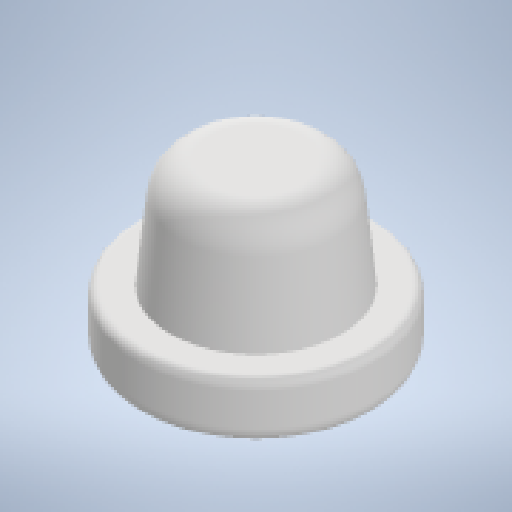
# Autodesk Inventor part: Part5
Saved by Autodesk Inventor 2025.1 (Build 291241000, 241)
## iProperties
Created: 2025-02-27
Part Number: Part5
Material: Generic
Document SubType Name: Modeling
Designer: santiago
Density: 1 g/cm^3
Appearance: Default
Author: santiago
Autodesk Inventor part; units mm, degrees
ref_plane "YZ Plane" through (0, 0, 0) normal (1, 0, 0) x (0, 1, 0)
ref_plane "XZ Plane" through (0, 0, 0) normal (0, 1, 0) x (-1, 0, 0)
ref_plane "XY Plane" through (0, 0, 0) normal (0, 0, 1) x (1, 0, 0)
sketch "Sketch1" plane through (0, 0, 0) normal (1, 0, 0) x (0, 1, 0)
  line L0 (10, 0) -> (10, 4.5)
  line L1 (10, 4.5) -> (2.5, 5.2)
  line L2 (2.5, 5.2) -> (2.5, 7.2)
  line L3 (2.5, 7.2) -> (0, 7.2)
  line L4 (0, 7.2) -> (0, 0)
  line L5 (10, 0) -> (0, 0)
  dimension "d0" = 4.5
  dimension "d1" = 10
  dimension "d2" = 2.5
  dimension "d3" = 2
  dimension "d5" = 7.2
  dimension "d6" = 5.2
  constraints: 12 end point, 2 perpendicular, 1 horizontal, 1 parallel, 1 vertical
  measures "d0" distance of L0.start L0.end
  measures "d1" distance between parallel lines of L4 L0
  measures "d2" distance between parallel lines of L4 L2
  measures "d3" distance of L1.end L2.end
  measures "d5" distance of L3.end L4.end
  measures "d6" distance from line of L5 L1.end
revolve "Revolution1" add sketch "Sketch1" angle 360 about axis through (0, 10, 0) along (0, -1, 0)
fillet "Fillet1" radius 2 1 edges at (0, 10, -4.5)
fillet "Fillet2" radius 0.5 1 edges at (0, 2.5, -7.2)
fillet "Fillet3" radius 1 1 edges at (0, 0, -7.2)
body "Solid1"
